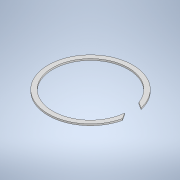
# Autodesk Inventor part: 65. Кольцо упорное подшипника
Saved by Autodesk Inventor 2021 (Build 250183000, 183)
## iProperties
Created: 2021-03-10
Part Number: 65. Кольцо упорное подшипника
Material: Типовые
Document SubType Name: Modeling
Designer: Данил
Density: 1 g/cm^3
Appearance: По умолчанию
Author: Данил
Autodesk Inventor part; units mm, degrees
ref_plane "YZ Plane" through (0, 0, 0) normal (1, 0, 0) x (0, 1, 0)
ref_plane "XZ Plane" through (0, 0, 0) normal (0, 1, 0) x (-1, 0, 0)
ref_plane "XY Plane" through (0, 0, 0) normal (0, 0, 1) x (1, 0, 0)
sketch "Эскиз1" plane through (0, 0, 0) normal (0, 0, 1) x (1, 0, 0)
  line L0 (0, 0.85) -> (0, -0.85)
  line L1 (40.5, 0.85) -> (40.5, -0.85)
  line L2 (40.5, -0.85) -> (45.4, -0.85)
  line L3 (45.4, -0.85) -> (45.4, 0.85)
  line L4 (45.4, 0.85) -> (40.5, 0.85)
  point P0 (0, 0)
  point P1 (0, 0)
  dimension "d0" = 1.7
  dimension "d1" = 81
  dimension "d2" = 4.9
  constraints: 10 end point, 3 perpendicular, 2 horizontal alignment, 2 vertical, 1 coincident, 1 midpoint
  measures "d0" distance of L0.start L0.end
  measures "d1" diameter of L1 L0
  measures "d2" distance between parallel lines of L3 L1
revolve "Вращение1" add sketch "Эскиз1" angle 360 about axis through (0, 0.85, 0) along (0, -1, 0)
sketch "Эскиз2" plane through (0, 0.85, 0) normal (0, 1, 0) x (1, 0, 0)
  line L0 (44.285, 10) -> (44.285, -10)
  circle A0 centre (0, 0) radius 45.4 projected
  line L1 (0, 0) -> (44.285, 10)
  line L2 (0, 0) -> (44.285, -10)
  line L3 (44.285, 10) -> (0, 37.9692)
  line L4 (44.285, -10) -> (23.2715, 23.2715)
  point P0 (0, 0)
  point P1 (44.285, 0)
  dimension "d4" = 20
  dimension "d6" = 45
  dimension "d7" = 45
  constraints: 10 end point, 1 horizontal alignment, 1 midpoint, 1 point on line, 1 vertical, 1 vertical alignment, 2 other
  measures "d4" distance of L0.start L0.end
  measures "d6" angle of L3 L1
  measures "d7" angle of L2 L4
extrude "Выдавливание1" cut sketch "Эскиз2" against normal through all contours A0 L0 | L0 L4 L1 | L1 L4 L3
